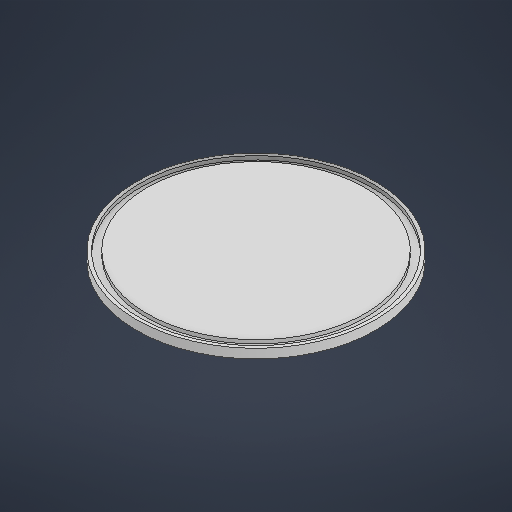
# Autodesk Inventor part: Base_Taza
Saved by Autodesk Inventor 2026 (Build 300175000, 175)
## iProperties
Created: 2025-06-27
Part Number: Base_Taza
Material: Genérico
Document SubType Name: Modeling
Designer: oscar
Density: 1 g/cm^3
Appearance: Valor por defecto
Author: oscar
Autodesk Inventor part; units mm, degrees
ref_plane "YZ Plane" through (0, 0, 0) normal (1, 0, 0) x (0, 1, 0)
ref_plane "XZ Plane" through (0, 0, 0) normal (0, 1, 0) x (-1, 0, 0)
ref_plane "XY Plane" through (0, 0, 0) normal (0, 0, 1) x (1, 0, 0)
sketch "Boceto1" plane through (0, 0, 0) normal (0, 1, 0) x (-1, 0, 0)
  circle A0 centre (0, 0) radius 62.75
  circle A1 centre (0, 0) radius 64.5
  circle A2 centre (0, 0) radius 58.85
  circle A3 centre (0, 0) radius 62.75
  circle A4 centre (0, 0) radius 58.85
  dimension "d0" = 125.5
  dimension "d1" = 129
  dimension "d2" = 117.7
  constraints: 5 centre point, 5 coincident, 2 concentric
  measures "d0" diameter of A0
  measures "d1" diameter of A1
  measures "d2" diameter of A2
extrude "Extrusión1" add sketch "Boceto1" along normal blind 5
sketch "Boceto3" plane through (0, 0, 0) normal (0, -1, 0) x (1, 0, 0)
  circle A0 centre (0, 0) radius 58.85
  circle A1 centre (0, 0) radius 62.75
  constraints: 2 centre point, 2 coincident
extrude "Extrusión2" add sketch "Boceto3" against normal blind 3
